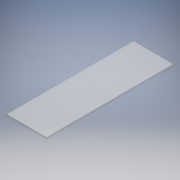
# Autodesk Inventor part: Vitre
Saved by Autodesk Inventor 2016 SP1 (Build 200210100, 210)
## iProperties
Created: 2016-10-04
Part Number: Vitre
Material: Verre
Document SubType Name: Modeling
Designer: dimercur
Density: 2.18 g/cm^3
Appearance: Transparent - Clair
Mass: 36022.3 g
Surface Area: 17376 cm^2
Volume: 16524 cm^3
Author: dimercur
Autodesk Inventor part; units mm, degrees
ref_plane "YZ Plane" through (0, 0, 0) normal (1, 0, 0) x (0, 1, 0)
ref_plane "XZ Plane" through (0, 0, 0) normal (0, 1, 0) x (-1, 0, 0)
ref_plane "XY Plane" through (0, 0, 0) normal (0, 0, 1) x (1, 0, 0)
sketch "Esquisse1" plane through (0, 0, 0) normal (0, 0, 1) x (1, 0, 0)
  line L0 (-222.2635, 460.8953) -> (287.7365, 460.8953)
  line L1 (287.7365, 460.8953) -> (287.7365, -1159.1047)
  line L2 (287.7365, -1159.1047) -> (-222.2635, -1159.1047)
  line L3 (-222.2635, -1159.1047) -> (-222.2635, 460.8953)
  point P0 (0, 0)
  dimension "d0" = 510
  dimension "d1" = 1620
  constraints: 8 end point, 2 parallel, 1 horizontal, 1 perpendicular
  measures "d0" distance of L0.start L0.end
  measures "d1" distance of L2.end L0.start
extrude "Extrusion1" add sketch "Esquisse1" along normal blind 20
